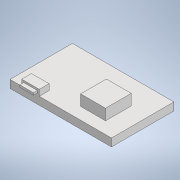
# Autodesk Inventor part: BMS
Saved by Autodesk Inventor 2020 (Build 240168000, 168)
## iProperties
Created: 2021-11-16
Part Number: BMS
Material: Generic
Document SubType Name: Modeling
Designer: mtkts
Density: 1 g/cm^3
Appearance: Default
Author: mtkts
Autodesk Inventor part; units mm, degrees
ref_plane "YZ Plane" through (0, 0, 0) normal (1, 0, 0) x (0, 1, 0)
ref_plane "XZ Plane" through (0, 0, 0) normal (0, 1, 0) x (-1, 0, 0)
ref_plane "XY Plane" through (0, 0, 0) normal (0, 0, 1) x (1, 0, 0)
sketch "Sketch1" plane through (0, 0, 0) normal (0, 1, 0) x (-1, 0, 0)
  line L0 (-13, 8) -> (13, 8)
  line L1 (13, 8) -> (13, -8)
  line L2 (13, -8) -> (-13, -8)
  line L3 (-13, -8) -> (-13, 8)
  line L4 (-13, 8) -> (13, -8) construction
  line L5 (13, 8) -> (-13, -8) construction
  point P0 (0, 0)
  dimension "d0" = 26
  dimension "d1" = 16
  constraints: 12 end point, 2 midpoint, 2 parallel, 1 horizontal, 1 perpendicular
  measures "d0" distance of L1.end L2.end
  measures "d1" distance of L0.end L1.end
extrude "Extrusion1" add sketch "Sketch1" along normal blind 2
sketch "Sketch2" plane through (0, 2, 0) normal (0, 1, 0) x (1, 0, 0)
  line L0 (13, -8) -> (13, 8) construction
  line L1 (13, 8) -> (-13, 8) construction
  line L2 (-13, 8) -> (-13, -8) construction
  line L3 (-13, -8) -> (13, -8) construction
  line L4 (-13, 8) -> (-13, -8) construction
  line L5 (-13, -8) -> (-10, -8) construction
  line L6 (-13, -8) -> (13, -8) construction
  line L7 (-10, -8) -> (-10, -5.5)
  line L8 (-10, -5.5) -> (-5.5, -5.5)
  line L9 (-5.5, -5.5) -> (-5.5, -8)
  line L10 (-5.5, -8) -> (-10, -8)
  point P0 (0, 0)
  dimension "d4" = 3
  dimension "d5" = 2.5
  dimension "d6" = 4.5
  constraints: 10 end point, 2 parallel, 2 perpendicular, 1 point on line
  measures "d4" distance of L2.end L5.end
  measures "d5" distance of L5.end L7.end
  measures "d6" distance of L7.end L8.end
extrude "Extrusion2" add sketch "Sketch2" along normal blind 1.55
sketch "Sketch3" plane through (-13, 0, 8) normal (0, 0, 1) x (1, 0, 0)
  line L0 (0, 0) -> (26, 0) construction
  line L1 (26, 0) -> (26, 2) construction
  line L2 (7.5, 2) -> (26, 2) construction
  line L3 (7.5, 2) -> (7.5, 3.55) construction
  line L4 (3, 3.55) -> (7.5, 3.55) construction
  line L5 (3, 2) -> (3, 3.55) construction
  line L6 (0, 2) -> (3, 2) construction
  line L7 (0, 0) -> (0, 2) construction
  line L8 (3, 3.55) -> (7.5, 3.55) construction
  line L9 (7.5, 3.55) -> (7.5, 2) construction
  line L10 (7.5, 2) -> (3, 2) construction
  line L11 (3, 2) -> (3, 3.55) construction
  line L12 (3.5, 2.5) -> (7, 2.5)
  line L13 (7, 2.5) -> (7, 3.05)
  line L14 (7, 3.05) -> (3.5, 3.05)
  line L15 (3.5, 3.05) -> (3.5, 2.5)
  point P0 (13, 0)
  dimension "d9" = 0.5
  constraints: 16 end point, 4 parallel, 2 perpendicular, 1 horizontal, 3 other
  measures "d9" distance between parallel lines of L10 L12
extrude "Extrusion3" add sketch "Sketch3" along normal blind 1
sketch "Sketch4" plane through (0, 2, 0) normal (0, 1, 0) x (1, 0, 0)
  line L0 (13, -8) -> (13, 8) construction
  line L1 (13, -8) -> (8.428, -8) construction
  line L2 (-13, -8) -> (13, -8) construction
  line L3 (8.428, -8) -> (8.428, -4.952) construction
  line L4 (8.428, -4.952) -> (2.0526, -4.952)
  line L5 (2.0526, -4.952) -> (2.0526, 1.652)
  line L6 (2.0526, 1.652) -> (8.428, 1.652)
  line L7 (8.428, 1.652) -> (8.428, -4.952)
  point P0 (0, 0)
  dimension "d12" = 4.572
  dimension "d13" = 3.048
  dimension "d14" = 6.3754
  dimension "d15" = 6.604
  constraints: 12 end point, 2 parallel, 2 perpendicular, 1 horizontal, 1 point on line
  measures "d12" distance of L0.start L1.end
  measures "d13" distance of L1.end L3.end
  measures "d14" distance of L5.end L6.end
  measures "d15" distance of L4.end L5.end
extrude "Extrusion4" add sketch "Sketch4" along normal blind 2.794
body "Solid1"
